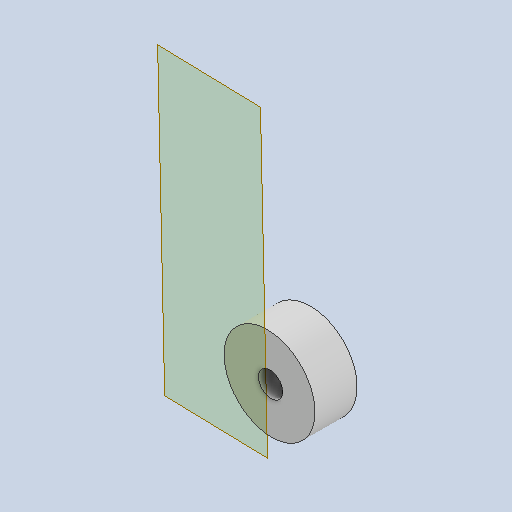
# Autodesk Inventor part: arm top
Saved by Autodesk Inventor 2024 (Build 280153000, 153)
## iProperties
Created: 2024-01-09
Part Number: arm top
Material: Generic
Document SubType Name: Modeling
Designer: MaartenGeorgesBuelen
Density: 1 g/cm^3
Appearance: Default
Author: MaartenGeorgesBuelen
Autodesk Inventor part; units mm, degrees
ref_plane "YZ Plane" through (0, 0, 0) normal (1, 0, 0) x (0, 1, 0)
ref_plane "XZ Plane" through (0, 0, 0) normal (0, 1, 0) x (-1, 0, 0)
ref_plane "Work Plane1" through (-1.9147, 139.6726, 27.3815) normal (0.0246, 0.0229, -0.9994) x (-0.9997, 0.0007, -0.0246)
sketch "Sketch1" plane through (-1.9147, 139.6726, 27.3815) normal (0.0246, 0.0229, -0.9994) x (-0.9997, 0.0007, -0.0246)
  circle A0 centre (-67.3467, -145.2099) radius 30.0404
  ellipse E0 centre (-68.007, -145.3208) end of major axis (-75.8787, -146.7707) minor radius 8 projected
  ellipse E1 centre (-68.007, -145.3208) end of major axis (-38.4484, -139.8763) minor radius 30.0404 (-97.2276, -138.2954) -> (-38.7864, -152.3461) ccw projected
  point P0 (-1.3436, -140.2639)
  constraints: 1 centre point, 3 other
ref_plane "Work Plane2" through (-4.7831, -40.7646, 0) normal (0, 0, 1) x (1, 0, 0)
extrude "Extrusion1" add sketch "Sketch1" along normal up to surface surface through (-4.7831, -40.7646, 0) normal (0, 0, 1)
body "Solid1"
